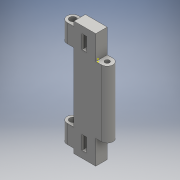
# Autodesk Inventor part: tracks
Saved by Autodesk Inventor 2016 (Build 200138000, 138)
## iProperties
Created: 2016-04-17
Part Number: tracks
Material: Generic
Document SubType Name: Modeling
Designer: Henrik Samuelsson
Density: 1 g/cm^3
Appearance: Default
Author: Henrik Samuelsson
Autodesk Inventor part; units mm, degrees
ref_plane "YZ Plane" through (0, 0, 0) normal (1, 0, 0) x (0, 1, 0)
ref_plane "XZ Plane" through (0, 0, 0) normal (0, 1, 0) x (-1, 0, 0)
ref_plane "XY Plane" through (0, 0, 0) normal (0, 0, 1) x (1, 0, 0)
sketch "Sketch1" plane through (0, 0, 0) normal (0, 1, 0) x (-1, 0, 0)
  line L0 (0, 0) -> (0, -10.5)
  line L1 (0, -10.5) -> (-4, -10.5)
  line L2 (-4, -10.5) -> (-4, -39.5)
  line L3 (-4, -39.5) -> (0, -39.5)
  line L4 (0, -39.5) -> (0, -50)
  line L5 (0, -50) -> (10.5, -50)
  line L6 (10.5, -50) -> (10.5, -48)
  line L7 (10.5, -48) -> (16, -48)
  line L8 (16, -48) -> (16, -40)
  line L9 (16, -40) -> (10.5, -40)
  line L10 (10.5, -40) -> (10.5, -10)
  line L11 (10.5, -10) -> (16, -10)
  line L12 (16, -10) -> (16, -2)
  line L13 (16, -2) -> (10.5, -2)
  line L14 (10.5, -2) -> (10.5, 0)
  line L15 (10.5, 0) -> (0, 0)
  line L16 (11, -3) -> (1, -3)
  line L17 (1, -3) -> (1, -9)
  line L18 (1, -9) -> (11, -9)
  line L19 (11, -9) -> (11, -3)
  line L20 (11, -41) -> (1, -41)
  line L21 (1, -41) -> (1, -47)
  line L22 (1, -47) -> (11, -47)
  line L23 (11, -47) -> (11, -41)
  dimension "d0" = 20
  dimension "d1" = 50
  dimension "d2" = 10.5
  dimension "d3" = 10.5
  dimension "d4" = 2
  dimension "d5" = 2
  dimension "d6" = 8
  dimension "d7" = 8
  dimension "d8" = 4
  dimension "d9" = 5.5
  dimension "d10" = 5.5
  dimension "d11" = 5.5
  dimension "d12" = 5.5
  dimension "d13" = 10
  dimension "d14" = 6
  dimension "d15" = 5
  dimension "d16" = 3
  dimension "d17" = 10
  dimension "d18" = 6
  dimension "d19" = 3
  constraints: 48 end point, 16 perpendicular, 4 parallel, 3 point on line, 2 horizontal, 1 vertical
  measures "d0" distance between parallel lines of L2 L12
  measures "d1" distance between parallel lines of L5 L15
  measures "d2" distance of L0.end L0.start
  measures "d3" distance of L4.end L3.end
  measures "d4" distance of L13.end L14.end
  measures "d5" distance of L5.end L6.end
  measures "d6" distance of L12.end L11.end
  measures "d7" distance of L7.end L8.end
  measures "d8" distance of L0.end L1.end
  measures "d9" distance of L13.end L12.end
  measures "d10" distance from line of L6 L7.end
  measures "d11" distance of L9.end L8.end
  measures "d12" distance from line of L10 L11.end
  measures "d13" distance of L17.end L18.end
  measures "d14" distance of L17.end L16.end
  measures "d15" distance from line of L2 L17.end
  measures "d16" distance from line of L15 L16.start
  measures "d17" distance of L21.end L22.end
  measures "d18" distance of L21.end L20.end
  measures "d19" distance between parallel lines of L5 L22
extrude "Extrusion1" add sketch "Sketch1" along normal blind 5
sketch "Sketch2" plane through (-11, 0, -9) normal (0, 0, 1) x (1, 0, 0)
  point P0 (11, 0)
ref_plane "Work Plane1" through (-6, 5, -9) normal (0, 0, 1) x (1, 0, 0)
sketch "Sketch4" plane through (-6, 5, -9) normal (0, 0, 1) x (1, 0, 0)
  line L0 (-5, -5) -> (5, -5) projected
  line L1 (5, -5) -> (-5, -5) projected
  line L2 (-5, -5) -> (5, -5) projected
  line L3 (5, -5) -> (-5, -5) projected
  line L4 (-4.5, -5) -> (6, -5) projected
  line L5 (-10, -5) -> (-4.5, -5) projected
  line L6 (-4.5, -5) -> (-10, -5) projected
  line L7 (-10, -5) -> (-4.5, -5) projected
  line L8 (-4.5, -5) -> (-10, -5) projected
  line L9 (6, -5) -> (-4.5, -5) projected
  line L10 (10, -5) -> (6, -5) projected
  line L11 (6, -5) -> (10, -5) projected
  line L12 (-5, 0) -> (5, 0) projected
  line L13 (5, 0) -> (-5, 0) projected
  line L14 (-5, 0) -> (5, 0) projected
  line L15 (5, 0) -> (-5, 0) projected
  line L16 (6, 0) -> (10, 0) projected
  line L17 (10, 0) -> (6, 0) projected
  line L18 (6, 0) -> (-4.5, 0) projected
  line L19 (-4.5, 0) -> (-10, 0) projected
  line L20 (-10, 0) -> (-4.5, 0) projected
  line L21 (-4.5, 0) -> (-10, 0) projected
  line L22 (-10, 0) -> (-4.5, 0) projected
  line L23 (-4.5, 0) -> (6, 0) projected
  line L24 (5, -5) -> (5, 0) projected
  line L25 (-5, -5) -> (-5, 0) projected
  line L26 (6, -5) -> (-4.5, -5) projected
  line L27 (-5, -5) -> (-5, 0) construction
  line L28 (-5, -5) -> (0, -5) construction
  line L29 (5, -5) -> (5, 0) projected
  line L30 (5, -5) -> (5, 0) construction
  line L31 (5, -5) -> (10, -5) construction
  line L32 (-5, 0) -> (-5, -5)
  line L33 (0, -5) -> (5, -5)
  line L34 (5, 0) -> (5, -5)
  line L35 (6, 0) -> (-4.5, 0) projected
  line L36 (-5, -5) -> (0, -5)
  line L37 (-5, -5) -> (-1, -5)
  line L38 (-1, -5) -> (-1, -4)
  line L39 (5, -5) -> (1, -5)
  line L40 (1, -5) -> (1, -4)
  line L41 (-5, -5) -> (-5, -4)
  line L42 (-5, -5) -> (-5, 0) projected
  line L43 (5, -5) -> (5, -4)
  arc A0 (5, 0) -> (1, -4) centre (5, -4) ccw
  arc A1 (-1, -4) -> (-5, 0) centre (-5, -4) ccw
  dimension "d26" = 90
  dimension "d28" = 90
  dimension "d48" = 4
  dimension "d49" = 1
  dimension "d50" = 4
  dimension "d51" = 1
  dimension "d52" = 4
  constraints: 28 end point, 4 coincident, 4 point on circle, 3 collinear, 3 perpendicular, 3 point on line, 2 centre point, 1 horizontal, 1 vertical, 5 other
  measures "d26" angle of L28 L27
  measures "d28" angle of L31 L30
  measures "d48" distance of L27.start L37.end
  measures "d49" distance of L37.end L38.end
  measures "d50" distance of L30.start L39.end
  measures "d51" distance of L39.end L40.end
  measures "d52" distance of L41.end L13.end
extrude "Extrusion2" add sketch "Sketch4" along normal blind 6 contours L25 A1 L38 L0 | L40 A0 L24 L0
sketch "Sketch6" plane through (-10.5, 0, -48) normal (0, 0, -1) x (-1, 0, 0)
  circle A0 centre (3, 2.5) radius 1.4
  line L0 (0, 0) -> (5.5, 0) projected
  line L1 (5.5, 0) -> (5.5, 5) projected
  line L2 (0, 5) -> (5.5, 5) projected
  line L3 (0, 0) -> (0, 5) projected
  point P0 (-10.5, 0)
  dimension "d34" = 2.5
  dimension "d35" = 2.5
  dimension "d47" = 2.8
  constraints: 1 centre point
  measures "d34" distance from line of L0 A0.centre
  measures "d35" distance from line of L1 A0.centre
  measures "d47" diameter of A0
extrude "Extrusion4" cut sketch "Sketch6" against normal through all contours A0
sketch "Sketch7" plane through (4, 0, -39.5) normal (0, 0, -1) x (-1, 0, 0)
  circle A0 centre (2.5, 2.5) radius 1
  line L0 (0, 5) -> (4, 5) projected
  line L1 (0, 0) -> (0, 5) projected
  point P0 (4, 0)
  dimension "d38" = 2
  dimension "d39" = 2.5
  dimension "d40" = 2.5
  constraints: 1 centre point
  measures "d38" diameter of A0
  measures "d39" distance from line of L1 A0.centre
  measures "d40" distance from line of L0 A0.centre
extrude "Extrusion5" cut sketch "Sketch7" against normal through all
sketch "Sketch8" plane through (-10.5, 0, -10) normal (0, 0, -1) x (-1, 0, 0)
  point P0 (-10.5, 0)
sketch "Sketch12" plane through (-1, 0, -41) normal (0, 0, -1) x (-1, 0, 0)
  line L0 (6, 1) -> (6, 0) projected
  line L1 (4, 0) -> (6, 0) projected
  line L2 (4, 0) -> (4, 1) projected
  arc A0 (4, 1) -> (0, 5) centre (0, 1) ccw projected
  line L3 (10, 5) -> (0, 5) projected
  arc A1 (10, 5) -> (6, 1) centre (10, 1) ccw projected
  arc A2 (4, 1) -> (0, 5) centre (0, 1) ccw
  arc A3 (10, 5) -> (6, 1) centre (10, 1) ccw
  line L4 (4, 0) -> (6, 0) projected
  line L5 (6, 1) -> (6, 0)
  line L6 (6, 0) -> (10, 0)
  line L7 (15, 0) -> (9.5, 0) projected
  line L8 (10, 5) -> (10, 0)
  line L9 (10, 0) -> (6, 0)
  line L10 (9.5, 0) -> (-1, 0) projected
  line L11 (4, 0) -> (0, 0)
  arc A4 (4, 1) -> (0, 5) centre (0, 1) ccw projected
  line L12 (0, 0) -> (0, 5)
  line L13 (4, 0) -> (4, 1) projected
  line L14 (4, 0) -> (4, 1)
  dimension "d54" = 5
  constraints: 14 end point, 4 point on circle, 3 vertical, 2 centre point, 2 coincident, 2 perpendicular, 2 point on line, 1 collinear
  measures "d54" distance of L6.end L3.start
extrude "Extrusion6" add sketch "Sketch12" along normal blind 6 contours A1 L8 L6 L0 | L10 L12 A0 L2
fillet "Fillet5" radius 2.5 6 edges at (-16, 5, -6) (-16, 5, -44) (4, 5, -25) (-16, 0, -6) (4, 0, -25) (-16, 0, -44)
sketch "Sketch13" plane through (0, 5, 0) normal (0, 1, 0) x (1, 0, 0)
  line L0 (-10.5, 0) -> (0, 0) projected
  line L1 (0, 0) -> (-1, 0)
  line L2 (-1, 0) -> (-1, 10.5)
  line L3 (-1, 10.5) -> (0, 10.5)
  line L4 (0, 10.5) -> (0, 0)
  line L5 (0, 39.5) -> (0, 50) projected
  line L6 (0, 39.5) -> (-1, 39.5)
  line L7 (-1, 39.5) -> (-1, 50)
  line L8 (-1, 50) -> (0, 50)
  line L9 (0, 50) -> (0, 39.5)
  dimension "d58" = 1
  constraints: 16 end point, 4 parallel, 2 horizontal, 2 perpendicular, 1 point on line
  measures "d58" distance of L2.end L3.end
extrude "Extrusion7" cut sketch "Sketch13" against normal through all
body "Solid1"
